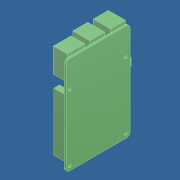
# Autodesk Inventor part: raspberry_pi_4B
Saved by Autodesk Inventor 2022.4 (Build 264492000, 492)
## iProperties
Created: 2023-07-26
Part Number: raspberry_pi_4B
Material: 一般
Document SubType Name: Modeling
Designer: 8326d
Density: 1 g/cm^3
Appearance: 滑らか - 濃い深緑
Author: 8326d
Autodesk Inventor part; units mm, degrees
(part 1 of 2)
ref_plane "YZ Plane" through (0, 0, 0) normal (1, 0, 0) x (0, 1, 0)
ref_plane "XZ Plane" through (0, 0, 0) normal (0, 1, 0) x (-1, 0, 0)
ref_plane "XY Plane" through (0, 0, 0) normal (0, 0, 1) x (1, 0, 0)
sketch "スケッチ1" plane through (0, 0, 0) normal (1, 0, 0) x (0, 1, 0)
  circle A0 centre (61.5, 3.5) radius 3
  circle A1 centre (3.5, 52.5) radius 1.35
  circle A2 centre (3.5, 52.5) radius 3
  circle A3 centre (3.5, 3.5) radius 1.35
  circle A4 centre (3.5, 3.5) radius 3
  circle A5 centre (61.5, 52.5) radius 1.35
  circle A6 centre (61.5, 52.5) radius 3
  circle A7 centre (61.5, 3.5) radius 1.35
  line L0 (3, 0) -> (82, 0)
  arc A8 (82, 0) -> (85, 3) centre (82, 3) ccw
  line L1 (85, 3) -> (85, 53)
  arc A9 (85, 53) -> (82, 56) centre (82, 53) ccw
  line L2 (82, 56) -> (3, 56)
  arc A10 (3, 56) -> (0, 53) centre (3, 53) ccw
  line L3 (0, 53) -> (0, 3)
  arc A11 (0, 3) -> (3, 0) centre (3, 3) ccw
  line L4 (33.225, 5.525) -> (34.375, 5.525)
  line L5 (34.375, 5.525) -> (34.375, 6.675)
  line L6 (34.375, 6.675) -> (33.225, 6.675)
  line L7 (33.225, 6.675) -> (33.225, 5.525)
  arc A12 (33.5, 6.5) -> (33.3, 6.5) centre (33.4, 6.5) ccw
  arc A13 (33.3, 6.5) -> (33.5, 6.5) centre (33.4, 6.5) ccw
  line L8 (6.6, 36.1) -> (17.4, 36.1)
  line L9 (17.4, 36.1) -> (17.4, 49.1)
  line L10 (17.4, 49.1) -> (6.6, 49.1)
  line L11 (6.6, 49.1) -> (6.6, 36.1)
  line L12 (6.8, 36.3) -> (17.2, 36.3)
  line L13 (17.2, 36.3) -> (17.2, 48.9)
  line L14 (17.2, 48.9) -> (6.8, 48.9)
  line L15 (6.8, 48.9) -> (6.8, 36.3)
  line L16 (6.6, 47.9) -> (6.8, 47.9)
  line L17 (6.6, 47.2) -> (6.8, 47.2)
  line L18 (36.4, -0.83) -> (36.4, 6.52)
  line L19 (36.4, 6.52) -> (42.6, 6.52)
  line L20 (42.6, 6.52) -> (42.6, -0.83)
  line L21 (42.6, -0.83) -> (36.4, -0.83)
  line L22 (36.4, -0.83) -> (35.9, -1.33)
  line L23 (35.9, -1.33) -> (35.9, -1.43)
  line L24 (35.9, -1.43) -> (43.1, -1.43)
  line L25 (43.1, -1.43) -> (43.1, -1.33)
  line L26 (43.1, -1.33) -> (42.6, -0.83)
  line L27 (22.9, -0.83) -> (22.9, 6.52)
  line L28 (22.9, 6.52) -> (29.1, 6.52)
  line L29 (29.1, 6.52) -> (29.1, -0.83)
  line L30 (29.1, -0.83) -> (22.9, -0.83)
  line L31 (22.9, -0.83) -> (22.4, -1.33)
  line L32 (22.4, -1.33) -> (22.4, -1.43)
  line L33 (22.4, -1.43) -> (29.6, -1.43)
  line L34 (29.6, -1.43) -> (29.6, -1.33)
  line L35 (29.6, -1.33) -> (29.1, -0.83)
  line L36 (8.95, 48.35) -> (8.15, 48.35)
  line L37 (8.15, 48.35) -> (8.15, 46.75)
  line L38 (8.15, 46.75) -> (8.95, 46.75)
  line L39 (8.95, 46.75) -> (8.95, 48.35)
  line L40 (8.7, 46.85) -> (8.7, 47.15)
  line L41 (8.7, 47.15) -> (8.4, 47.15)
  line L42 (8.4, 47.15) -> (8.4, 46.85)
  line L43 (8.4, 46.85) -> (8.7, 46.85)
  line L44 (68.4, 17.3) -> (68.4, 18.5)
  line L45 (68.4, 18.5) -> (66.4, 18.5)
  line L46 (66.4, 18.5) -> (66.4, 17.3)
  line L47 (66.4, 17.3) -> (68.4, 17.3)
  line L48 (68, 17.3) -> (68, 18.5)
  line L49 (66.8, 17.3) -> (66.8, 18.5)
  line L50 (51.4, 18.6) -> (54.4, 18.6)
  line L51 (54.4, 18.6) -> (54.4, 20.6)
  line L52 (54.4, 20.6) -> (51.4, 20.6)
  line L53 (51.4, 20.6) -> (51.4, 18.6)
  arc A14 (51.8414, 20.3) -> (51.5586, 20.3) centre (51.7, 20.3) ccw
  arc A15 (51.5586, 20.3) -> (51.8414, 20.3) centre (51.7, 20.3) ccw
  line L54 (50.5, 16.9) -> (50.5, 13.9)
  line L55 (50.5, 13.9) -> (52.5, 13.9)
  line L56 (52.5, 13.9) -> (52.5, 16.9)
  line L57 (52.5, 16.9) -> (50.5, 16.9)
  arc A16 (52.3414, 16.6) -> (52.0586, 16.6) centre (52.2, 16.6) ccw
  arc A17 (52.0586, 16.6) -> (52.3414, 16.6) centre (52.2, 16.6) ccw
  line L58 (39.05, 40) -> (39.05, 39.6)
  line L59 (39.05, 39.6) -> (39.45, 40)
  line L60 (39.45, 40) -> (39.05, 40)
  line L61 (39.05, 25) -> (50.55, 25)
  line L62 (50.55, 25) -> (50.55, 40)
  line L63 (50.55, 40) -> (39.05, 40)
  line L64 (39.05, 40) -> (39.05, 25)
  line L65 (68.4, 15.3) -> (68.4, 16.5)
  line L66 (68.4, 16.5) -> (66.4, 16.5)
  line L67 (66.4, 16.5) -> (66.4, 15.3)
  line L68 (66.4, 15.3) -> (68.4, 15.3)
  line L69 (68, 15.3) -> (68, 16.5)
  line L70 (66.8, 15.3) -> (66.8, 16.5)
  line L71 (3.8, 16.3) -> (2.6, 16.3)
  line L72 (2.6, 16.3) -> (2.6, 14.3)
  line L73 (2.6, 14.3) -> (3.8, 14.3)
  line L74 (3.8, 14.3) -> (3.8, 16.3)
  line L75 (3.8, 15.9) -> (2.6, 15.9)
  line L76 (3.8, 14.7) -> (2.6, 14.7)
  line L77 (6.875, -1.25) -> (15.525, -1.25)
  line L78 (15.525, -1.25) -> (15.525, 6.15)
  line L79 (15.525, 6.15) -> (6.875, 6.15)
  line L80 (6.875, 6.15) -> (6.875, -1.25)
  line L81 (12.9, 15.1) -> (12.9, 17.1)
  line L82 (12.9, 17.1) -> (13.9, 18.1)
  line L83 (13.9, 18.1) -> (15.9, 18.1)
  line L84 (15.9, 18.1) -> (16.9, 17.1)
  line L85 (16.9, 17.1) -> (16.9, 15.1)
  line L86 (16.9, 15.1) -> (15.9, 14.1)
  line L87 (15.9, 14.1) -> (13.9, 14.1)
  line L88 (13.9, 14.1) -> (12.9, 15.1)
  line L89 (69.85, 29.75) -> (69.85, 37.05)
  line L90 (69.85, 37.05) -> (65.55, 37.05)
  line L91 (65.55, 37.05) -> (65.55, 29.75)
  line L92 (65.55, 29.75) -> (69.85, 29.75)
  line L93 (68.9, 29.75) -> (68.9, 31.05)
  line L94 (68.9, 31.05) -> (66.5, 31.05)
  line L95 (66.5, 31.05) -> (66.5, 29.75)
  line L96 (68.9, 37.05) -> (68.9, 35.75)
  line L97 (68.9, 35.75) -> (66.5, 35.75)
  line L98 (66.5, 35.75) -> (66.5, 37.05)
  line L99 (65.85, 30.25) -> (66.2, 30.25)
  line L100 (66, 30.05) -> (66, 30.45)
  line L101 (65.85, 30.25) -> (65.8, 30.25)
  line L102 (65.55, 30.75) -> (69.85, 30.75)
  line L103 (69.85, 30.75) -> (69.85, 31.45)
  line L104 (69.85, 31.45) -> (65.55, 31.45)
  line L105 (65.55, 31.45) -> (65.55, 30.75)
  line L106 (88, 37.995) -> (88, 53.505)
  line L107 (88, 53.505) -> (66.65, 53.505)
  line L108 (66.65, 53.505) -> (66.65, 37.995)
  line L109 (66.65, 37.995) -> (88, 37.995)
  line L110 (45.05, 0.3) -> (47.9, 0.3)
  line L111 (47.9, 0.3) -> (47.9, 3.7)
  line L112 (47.9, 3.7) -> (49, 4.8)
  line L113 (49, 4.8) -> (49, 18.2)
  line L114 (49, 18.2) -> (47.85, 19.35)
  line L115 (47.85, 19.35) -> (47.85, 22.7)
  line L116 (47.85, 22.7) -> (45.05, 22.7)
  line L117 (45.05, 22.7) -> (45.05, 0.3)
  line L118 (45.05, 3.5) -> (45.95, 3.5)
  line L119 (45.95, 3.5) -> (45.95, 19.5)
  line L120 (45.95, 19.5) -> (45.05, 19.5)
  line L121 (5.45, 39.2) -> (2.6, 39.2)
  line L122 (2.6, 39.2) -> (2.6, 35.8)
  line L123 (2.6, 35.8) -> (1.5, 34.7)
  line L124 (1.5, 34.7) -> (1.5, 21.3)
  line L125 (1.5, 21.3) -> (2.65, 20.15)
  line L126 (2.65, 20.15) -> (2.65, 16.8)
  line L127 (2.65, 16.8) -> (5.45, 16.8)
  line L128 (5.45, 16.8) -> (5.45, 39.2)
  line L129 (5.45, 36) -> (4.55, 36)
  line L130 (4.55, 36) -> (4.55, 20)
  line L131 (4.55, 20) -> (5.45, 20)
  line L132 (50.5, 0) -> (57.5, 0)
  line L133 (57.5, 0) -> (57.5, 12.5)
  line L134 (57.5, 12.5) -> (50.5, 12.5)
  line L135 (50.5, 12.5) -> (50.5, 0)
  line L136 (51, -2.5) -> (57, -2.5)
  line L137 (57, -2.5) -> (57, 0)
  line L138 (57, 0) -> (51, 0)
  line L139 (51, 0) -> (51, -2.5)
  line L140 (59.9, 18.4) -> (59.9, 16)
  line L141 (59.9, 16) -> (63.1, 16)
  line L142 (63.1, 16) -> (63.1, 18.4)
  line L143 (63.1, 18.4) -> (59.9, 18.4)
  line L144 (59.9, 18.4) -> (59.9, 18.3)
  line L145 (60, 18.3) -> (63, 18.3)
  line L146 (63, 18.3) -> (63, 16.1)
  line L147 (63, 16.1) -> (60, 16.1)
  line L148 (60, 16.1) -> (60, 18.3)
  arc A18 (60.4414, 16.4) -> (60.1586, 16.4) centre (60.3, 16.4) ccw
  arc A19 (60.1586, 16.4) -> (60.4414, 16.4) centre (60.3, 16.4) ccw
  line L149 (2.7, 47.25) -> (2.7, 49.85)
  line L150 (2.7, 49.85) -> (0.1, 49.85)
  line L151 (0.1, 49.85) -> (0.1, 47.25)
  line L152 (0.1, 47.25) -> (2.7, 47.25)
  line L153 (2.7, 48.85) -> (3, 48.85)
  line L154 (3, 48.85) -> (3, 48.25)
  line L155 (3, 48.25) -> (2.7, 48.25)
  arc A20 (2.322, 48.55) -> (0.478, 48.55) centre (1.4, 48.55) ccw
  arc A21 (0.478, 48.55) -> (2.322, 48.55) centre (1.4, 48.55) ccw
  arc A22 (1.6, 48.55) -> (1.2, 48.55) centre (1.4, 48.55) ccw
  arc A23 (1.2, 48.55) -> (1.6, 48.55) centre (1.4, 48.55) ccw
  line L156 (2.3, 47.25) -> (2.3, 47.05)
  line L157 (2.3, 47.05) -> (0.5, 47.05)
  line L158 (0.5, 47.05) -> (0.5, 47.25)
  line L159 (0.5, 49.85) -> (0.5, 50.05)
  line L160 (0.5, 50.05) -> (2.3, 50.05)
  line L161 (2.3, 50.05) -> (2.3, 49.85)
  line L162 (9.05, 43.2) -> (9.05, 42.9)
  line L163 (8.65, 42.9) -> (8.65, 43.2)
  line L164 (8.55, 42.9) -> (9.15, 42.9)
  line L165 (9.15, 42.9) -> (9.15, 43.2)
  line L166 (9.15, 43.2) -> (8.55, 43.2)
  line L167 (8.55, 43.2) -> (8.55, 42.9)
  arc A24 (8.8, 43.05) -> (8.7, 43.05) centre (8.75, 43.05) ccw
  arc A25 (8.7, 43.05) -> (8.8, 43.05) centre (8.75, 43.05) ccw
  line L168 (9.55, 43.8) -> (9.55, 43.5)
  line L169 (9.15, 43.5) -> (9.15, 43.8)
  line L170 (9.05, 43.5) -> (9.65, 43.5)
  line L171 (9.65, 43.5) -> (9.65, 43.8)
  line L172 (9.65, 43.8) -> (9.05, 43.8)
  line L173 (9.05, 43.8) -> (9.05, 43.5)
  arc A26 (9.3, 43.65) -> (9.2, 43.65) centre (9.25, 43.65) ccw
  arc A27 (9.2, 43.65) -> (9.3, 43.65) centre (9.25, 43.65) ccw
  line L174 (8.7, 43.7) -> (8.4, 43.7)
  line L175 (8.4, 44.1) -> (8.7, 44.1)
  line L176 (8.4, 44.2) -> (8.4, 43.6)
  line L177 (8.4, 43.6) -> (8.7, 43.6)
  line L178 (8.7, 43.6) -> (8.7, 44.2)
  line L179 (8.7, 44.2) -> (8.4, 44.2)
  arc A28 (8.6, 44) -> (8.5, 44) centre (8.55, 44) ccw
  arc A29 (8.5, 44) -> (8.6, 44) centre (8.55, 44) ccw
  line L180 (11.95, 44.75) -> (11.65, 44.75)
  line L181 (11.65, 45.15) -> (11.95, 45.15)
  line L182 (11.65, 45.25) -> (11.65, 44.65)
  line L183 (11.65, 44.65) -> (11.95, 44.65)
  line L184 (11.95, 44.65) -> (11.95, 45.25)
  line L185 (11.95, 45.25) -> (11.65, 45.25)
  arc A30 (11.85, 45.05) -> (11.75, 45.05) centre (11.8, 45.05) ccw
  arc A31 (11.75, 45.05) -> (11.85, 45.05) centre (11.8, 45.05) ccw
  line L186 (7.55, 38.35) -> (8.85, 38.35)
  line L187 (8.85, 38.35) -> (8.85, 40.05)
  line L188 (8.85, 40.05) -> (7.55, 40.05)
  line L189 (7.55, 40.05) -> (7.55, 38.35)
  arc A32 (8.05, 39.7) -> (7.65, 39.7) centre (7.85, 39.7) ccw
  arc A33 (7.65, 39.7) -> (8.05, 39.7) centre (7.85, 39.7) ccw
  line L190 (8.15, 46.175) -> (8.275, 46.3)
  line L191 (8.275, 46.3) -> (9.25, 46.3)
  line L192 (9.25, 46.3) -> (9.25, 45.2)
  line L193 (9.25, 45.2) -> (8.15, 45.2)
  line L194 (8.15, 45.2) -> (8.15, 46.175)
  line L195 (88, 2.43) -> (70.3, 2.43)
  line L196 (70.3, 2.43) -> (70.3, 15.57)
  line L197 (70.3, 15.57) -> (88, 15.57)
  line L198 (88, 15.57) -> (88, 1.65)
  line L199 (88, 1.65) -> (87.5, 1.65)
  line L200 (87.5, 1.65) -> (87.5, 2.43)
  line L201 (88, 15.57) -> (88, 16.35)
  line L202 (88, 16.35) -> (87.5, 16.35)
  line L203 (87.5, 16.35) -> (87.5, 15.57)
  line L204 (15.8, 19.5) -> (8.2, 19.5)
  line L205 (8.2, 19.5) -> (8.2, 21.5)
  line L206 (8.2, 21.5) -> (15.8, 21.5)
  line L207 (15.8, 21.5) -> (15.8, 19.5)
  line L208 (62.7, 14.75) -> (62.7, 14.25)
  line L209 (62.7, 14.25) -> (63.7, 14.25)
  line L210 (63.7, 14.25) -> (63.7, 14.75)
  line L211 (63.7, 14.75) -> (62.7, 14.75)
  line L212 (62.95, 14.25) -> (62.95, 14.75)
  line L213 (63.45, 14.25) -> (63.45, 14.75)
  line L214 (38.7, 43.25) -> (38.7, 42.75)
  line L215 (38.7, 42.75) -> (39.7, 42.75)
  line L216 (39.7, 42.75) -> (39.7, 43.25)
  line L217 (39.7, 43.25) -> (38.7, 43.25)
  line L218 (38.95, 42.75) -> (38.95, 43.25)
  line L219 (39.45, 42.75) -> (39.45, 43.25)
  line L220 (52.4, 18.15) -> (52.4, 17.65)
  line L221 (52.4, 17.65) -> (53.4, 17.65)
  line L222 (53.4, 17.65) -> (53.4, 18.15)
  line L223 (53.4, 18.15) -> (52.4, 18.15)
  line L224 (52.65, 17.65) -> (52.65, 18.15)
  line L225 (53.15, 17.65) -> (53.15, 18.15)
  line L226 (56.45, 32.6) -> (56.95, 32.6)
  line L227 (56.95, 32.6) -> (56.95, 33.6)
  line L228 (56.95, 33.6) -> (56.45, 33.6)
  line L229 (56.45, 33.6) -> (56.45, 32.6)
  line L230 (56.95, 32.85) -> (56.45, 32.85)
  line L231 (56.95, 33.35) -> (56.45, 33.35)
  line L232 (10.4, 8.25) -> (10.4, 7.75)
  line L233 (10.4, 7.75) -> (11.4, 7.75)
  line L234 (11.4, 7.75) -> (11.4, 8.25)
  line L235 (11.4, 8.25) -> (10.4, 8.25)
  line L236 (10.65, 7.75) -> (10.65, 8.25)
  line L237 (11.15, 7.75) -> (11.15, 8.25)
  line L238 (8.5, 8.25) -> (8.5, 7.75)
  line L239 (8.5, 7.75) -> (9.5, 7.75)
  line L240 (9.5, 7.75) -> (9.5, 8.25)
  line L241 (9.5, 8.25) -> (8.5, 8.25)
  line L242 (8.75, 7.75) -> (8.75, 8.25)
  line L243 (9.25, 7.75) -> (9.25, 8.25)
  line L244 (67.9, 19.25) -> (67.9, 19.75)
  line L245 (67.9, 19.75) -> (66.9, 19.75)
  line L246 (66.9, 19.75) -> (66.9, 19.25)
  line L247 (66.9, 19.25) -> (67.9, 19.25)
  line L248 (67.65, 19.75) -> (67.65, 19.25)
  line L249 (67.15, 19.75) -> (67.15, 19.25)
  line L250 (66.75, 2.4) -> (67.25, 2.4)
  line L251 (67.25, 2.4) -> (67.25, 3.4)
  line L252 (67.25, 3.4) -> (66.75, 3.4)
  line L253 (66.75, 3.4) -> (66.75, 2.4)
  line L254 (67.25, 2.65) -> (66.75, 2.65)
  line L255 (67.25, 3.15) -> (66.75, 3.15)
  line L256 (69.25, 3.4) -> (68.75, 3.4)
  line L257 (68.75, 3.4) -> (68.75, 2.4)
  line L258 (68.75, 2.4) -> (69.25, 2.4)
  line L259 (69.25, 2.4) -> (69.25, 3.4)
  line L260 (68.75, 3.15) -> (69.25, 3.15)
  line L261 (68.75, 2.65) -> (69.25, 2.65)
  line L262 (67.75, 2.4) -> (68.25, 2.4)
  line L263 (68.25, 2.4) -> (68.25, 3.4)
  line L264 (68.25, 3.4) -> (67.75, 3.4)
  line L265 (67.75, 3.4) -> (67.75, 2.4)
  line L266 (68.25, 2.65) -> (67.75, 2.65)
  line L267 (68.25, 3.15) -> (67.75, 3.15)
  line L268 (57.45, 16.7) -> (56.95, 16.7)
  line L269 (56.95, 16.7) -> (56.95, 15.7)
  line L270 (56.95, 15.7) -> (57.45, 15.7)
  line L271 (57.45, 15.7) -> (57.45, 16.7)
  line L272 (56.95, 16.45) -> (57.45, 16.45)
  line L273 (56.95, 15.95) -> (57.45, 15.95)
  line L274 (57.45, 14.8) -> (56.95, 14.8)
  line L275 (56.95, 14.8) -> (56.95, 13.8)
  line L276 (56.95, 13.8) -> (57.45, 13.8)
  line L277 (57.45, 13.8) -> (57.45, 14.8)
  line L278 (56.95, 14.55) -> (57.45, 14.55)
  line L279 (56.95, 14.05) -> (57.45, 14.05)
  line L280 (62.05, 7.5) -> (62.55, 7.5)
  line L281 (62.55, 7.5) -> (62.55, 8.5)
  line L282 (62.55, 8.5) -> (62.05, 8.5)
  line L283 (62.05, 8.5) -> (62.05, 7.5)
  line L284 (62.55, 7.75) -> (62.05, 7.75)
  line L285 (62.55, 8.25) -> (62.05, 8.25)
  line L286 (54.25, 16.7) -> (53.75, 16.7)
  line L287 (53.75, 16.7) -> (53.75, 15.7)
  line L288 (53.75, 15.7) -> (54.25, 15.7)
  line L289 (54.25, 15.7) -> (54.25, 16.7)
  line L290 (53.75, 16.45) -> (54.25, 16.45)
  line L291 (53.75, 15.95) -> (54.25, 15.95)
  line L292 (54.25, 14.8) -> (53.75, 14.8)
  line L293 (53.75, 14.8) -> (53.75, 13.8)
  line L294 (53.75, 13.8) -> (54.25, 13.8)
  line L295 (54.25, 13.8) -> (54.25, 14.8)
  line L296 (53.75, 14.55) -> (54.25, 14.55)
  line L297 (53.75, 14.05) -> (54.25, 14.05)
  line L298 (62.55, 10.6) -> (62.05, 10.6)
  line L299 (62.05, 10.6) -> (62.05, 9.6)
  line L300 (62.05, 9.6) -> (62.55, 9.6)
  line L301 (62.55, 9.6) -> (62.55, 10.6)
  line L302 (62.05, 10.35) -> (62.55, 10.35)
  line L303 (62.05, 9.85) -> (62.55, 9.85)
  line L304 (69.85, 11) -> (69.35, 11)
  line L305 (69.35, 11) -> (69.35, 10)
  line L306 (69.35, 10) -> (69.85, 10)
  line L307 (69.85, 10) -> (69.85, 11)
  line L308 (69.35, 10.75) -> (69.85, 10.75)
  line L309 (69.35, 10.25) -> (69.85, 10.25)
  line L310 (69.85, 9) -> (69.35, 9)
  line L311 (69.35, 9) -> (69.35, 8)
  line L312 (69.35, 8) -> (69.85, 8)
  line L313 (69.85, 8) -> (69.85, 9)
  line L314 (69.35, 8.75) -> (69.85, 8.75)
  line L315 (69.35, 8.25) -> (69.85, 8.25)
  line L316 (28.75, 23.1) -> (28.25, 23.1)
  line L317 (28.25, 23.1) -> (28.25, 22.1)
  line L318 (28.25, 22.1) -> (28.75, 22.1)
  line L319 (28.75, 22.1) -> (28.75, 23.1)
  line L320 (28.25, 22.85) -> (28.75, 22.85)
  line L321 (28.25, 22.35) -> (28.75, 22.35)
  line L322 (18.2, 48.85) -> (18.2, 48.35)
  line L323 (18.2, 48.35) -> (19.2, 48.35)
  line L324 (19.2, 48.35) -> (19.2, 48.85)
  line L325 (19.2, 48.85) -> (18.2, 48.85)
  line L326 (18.45, 48.35) -> (18.45, 48.85)
  line L327 (18.95, 48.35) -> (18.95, 48.85)
  line L328 (18.2, 47.85) -> (18.2, 47.35)
  line L329 (18.2, 47.35) -> (19.2, 47.35)
  line L330 (19.2, 47.35) -> (19.2, 47.85)
  line L331 (19.2, 47.85) -> (18.2, 47.85)
  line L332 (18.45, 47.35) -> (18.45, 47.85)
  line L333 (18.95, 47.35) -> (18.95, 47.85)
  line L334 (62.5, 35.25) -> (62.5, 34.75)
  line L335 (62.5, 34.75) -> (63.5, 34.75)
  line L336 (63.5, 34.75) -> (63.5, 35.25)
  line L337 (63.5, 35.25) -> (62.5, 35.25)
  line L338 (62.75, 34.75) -> (62.75, 35.25)
  line L339 (63.25, 34.75) -> (63.25, 35.25)
  line L340 (58.9, 31.9) -> (59.4, 31.9)
  line L341 (59.4, 31.9) -> (59.4, 32.9)
  line L342 (59.4, 32.9) -> (58.9, 32.9)
  line L343 (58.9, 32.9) -> (58.9, 31.9)
  line L344 (59.4, 32.15) -> (58.9, 32.15)
  line L345 (59.4, 32.65) -> (58.9, 32.65)
  line L346 (5.6, 12.5) -> (4, 12.5)
  line L347 (4, 12.5) -> (4, 13.3)
  line L348 (4, 13.3) -> (5.6, 13.3)
  line L349 (5.6, 13.3) -> (5.6, 12.5)
  line L350 (5.2, 13.3) -> (5.2, 12.5)
  line L351 (4.3, 13.3) -> (4.3, 12.5)
  line L352 (14.2, 11.9) -> (15.8, 11.9)
  line L353 (15.8, 11.9) -> (15.8, 11.1)
  line L354 (15.8, 11.1) -> (14.2, 11.1)
  line L355 (14.2, 11.1) -> (14.2, 11.9)
  line L356 (14.6, 11.1) -> (14.6, 11.9)
  line L357 (15.5, 11.1) -> (15.5, 11.9)
  line L358 (15.7, 8.5) -> (15.7, 10.1)
  line L359 (15.7, 10.1) -> (16.5, 10.1)
  line L360 (16.5, 10.1) -> (16.5, 8.5)
  line L361 (16.5, 8.5) -> (15.7, 8.5)
  line L362 (16.5, 8.9) -> (15.7, 8.9)
  line L363 (16.5, 9.8) -> (15.7, 9.8)
  line L364 (5.6, 11.1) -> (4, 11.1)
  line L365 (4, 11.1) -> (4, 11.9)
  line L366 (4, 11.9) -> (5.6, 11.9)
  line L367 (5.6, 11.9) -> (5.6, 11.1)
  line L368 (5.2, 11.9) -> (5.2, 11.1)
  line L369 (4.3, 11.9) -> (4.3, 11.1)
  line L370 (14.2, 13.3) -> (15.8, 13.3)
  line L371 (15.8, 13.3) -> (15.8, 12.5)
  line L372 (15.8, 12.5) -> (14.2, 12.5)
  line L373 (14.2, 12.5) -> (14.2, 13.3)
  line L374 (14.6, 12.5) -> (14.6, 13.3)
  line L375 (15.5, 12.5) -> (15.5, 13.3)
  line L376 (7.5, 16.6) -> (9.1, 16.6)
  line L377 (9.1, 16.6) -> (9.1, 15.8)
  line L378 (9.1, 15.8) -> (7.5, 15.8)
  line L379 (7.5, 15.8) -> (7.5, 16.6)
  line L380 (7.9, 15.8) -> (7.9, 16.6)
  line L381 (8.8, 15.8) -> (8.8, 16.6)
  line L382 (61, 33.4) -> (61, 31.8)
  line L383 (61, 31.8) -> (60.2, 31.8)
  line L384 (60.2, 31.8) -> (60.2, 33.4)
  line L385 (60.2, 33.4) -> (61, 33.4)
  line L386 (60.2, 33) -> (61, 33)
  line L387 (60.2, 32.1) -> (61, 32.1)
  line L388 (58.3, 33.4) -> (58.3, 31.8)
  line L389 (58.3, 31.8) -> (57.5, 31.8)
  line L390 (57.5, 31.8) -> (57.5, 33.4)
  line L391 (57.5, 33.4) -> (58.3, 33.4)
  line L392 (57.5, 33) -> (58.3, 33)
  line L393 (57.5, 32.1) -> (58.3, 32.1)
  line L394 (64.7, 8.2) -> (64.7, 9.8)
  line L395 (64.7, 9.8) -> (65.5, 9.8)
  line L396 (65.5, 9.8) -> (65.5, 8.2)
  line L397 (65.5, 8.2) -> (64.7, 8.2)
  line L398 (65.5, 8.6) -> (64.7, 8.6)
  line L399 (65.5, 9.5) -> (64.7, 9.5)
  line L400 (15.05, 41.65) -> (15.05, 41.15)
  line L401 (15.05, 41.15) -> (16.05, 41.15)
  line L402 (16.05, 41.15) -> (16.05, 41.65)
  line L403 (16.05, 41.65) -> (15.05, 41.65)
  line L404 (15.3, 41.15) -> (15.3, 41.65)
  line L405 (15.8, 41.15) -> (15.8, 41.65)
  line L406 (11.85, 38.05) -> (11.35, 38.05)
  line L407 (11.35, 38.05) -> (11.35, 37.05)
  line L408 (11.35, 37.05) -> (11.85, 37.05)
  line L409 (11.85, 37.05) -> (11.85, 38.05)
  line L410 (11.35, 37.8) -> (11.85, 37.8)
  line L411 (11.35, 37.3) -> (11.85, 37.3)
  line L412 (14.4, 38.05) -> (13.9, 38.05)
  line L413 (13.9, 38.05) -> (13.9, 37.05)
  line L414 (13.9, 37.05) -> (14.4, 37.05)
  line L415 (14.4, 37.05) -> (14.4, 38.05)
  line L416 (13.9, 37.8) -> (14.4, 37.8)
  line L417 (13.9, 37.3) -> (14.4, 37.3)
  line L418 (13.55, 38.05) -> (13.05, 38.05)
  line L419 (13.05, 38.05) -> (13.05, 37.05)
  line L420 (13.05, 37.05) -> (13.55, 37.05)
  line L421 (13.55, 37.05) -> (13.55, 38.05)
  line L422 (13.05, 37.8) -> (13.55, 37.8)
  line L423 (13.05, 37.3) -> (13.55, 37.3)
  line L424 (12.7, 38.05) -> (12.2, 38.05)
  line L425 (12.2, 38.05) -> (12.2, 37.05)
  line L426 (12.2, 37.05) -> (12.7, 37.05)
  line L427 (12.7, 37.05) -> (12.7, 38.05)
  line L428 (12.2, 37.8) -> (12.7, 37.8)
  line L429 (12.2, 37.3) -> (12.7, 37.3)
  line L430 (14.8, 37.95) -> (15.3, 37.95)
  line L431 (15.3, 37.95) -> (15.3, 38.95)
  line L432 (15.3, 38.95) -> (14.8, 38.95)
  line L433 (14.8, 38.95) -> (14.8, 37.95)
  line L434 (15.3, 38.2) -> (14.8, 38.2)
  line L435 (15.3, 38.7) -> (14.8, 38.7)
  line L436 (10.05, 44.4) -> (10.05, 44.9)
  line L437 (10.05, 44.9) -> (9.05, 44.9)
  line L438 (9.05, 44.9) -> (9.05, 44.4)
  line L439 (9.05, 44.4) -> (10.05, 44.4)
  line L440 (9.8, 44.9) -> (9.8, 44.4)
  line L441 (9.3, 44.9) -> (9.3, 44.4)
  line L442 (12.55, 8.4) -> (12.05, 8.4)
  line L443 (12.05, 8.4) -> (12.05, 7.4)
  line L444 (12.05, 7.4) -> (12.55, 7.4)
  line L445 (12.55, 7.4) -> (12.55, 8.4)
  line L446 (12.05, 8.15) -> (12.55, 8.15)
  line L447 (12.05, 7.65) -> (12.55, 7.65)
  line L448 (11.2, 44.75) -> (10.9, 44.75)
  line L449 (10.9, 45.15) -> (11.2, 45.15)
  line L450 (10.9, 45.25) -> (10.9, 44.65)
  line L451 (10.9, 44.65) -> (11.2, 44.65)
  line L452 (11.2, 44.65) -> (11.2, 45.25)
  line L453 (11.2, 45.25) -> (10.9, 45.25)
  line L454 (10.75, 48.05) -> (10.75, 48.35)
  line L455 (11.15, 48.35) -> (11.15, 48.05)
  line L456 (11.25, 48.35) -> (10.65, 48.35)
  line L457 (10.65, 48.35) -> (10.65, 48.05)
  line L458 (10.65, 48.05) -> (11.25, 48.05)
  line L459 (11.25, 48.05) -> (11.25, 48.35)
  line L460 (3.15, 42.4) -> (2.85, 42.4)
  line L461 (2.85, 42.8) -> (3.15, 42.8)
  line L462 (2.85, 42.9) -> (2.85, 42.3)
  line L463 (2.85, 42.3) -> (3.15, 42.3)
  line L464 (3.15, 42.3) -> (3.15, 42.9)
  line L465 (3.15, 42.9) -> (2.85, 42.9)
  line L466 (3.15, 41.1) -> (2.85, 41.1)
  line L467 (2.85, 41.5) -> (3.15, 41.5)
  line L468 (2.85, 41.6) -> (2.85, 41)
  line L469 (2.85, 41) -> (3.15, 41)
  line L470 (3.15, 41) -> (3.15, 41.6)
  line L471 (3.15, 41.6) -> (2.85, 41.6)
  line L472 (0.8, 42.4) -> (0.5, 42.4)
  line L473 (0.5, 42.8) -> (0.8, 42.8)
  line L474 (0.5, 42.9) -> (0.5, 42.3)
  line L475 (0.5, 42.3) -> (0.8, 42.3)
  line L476 (0.8, 42.3) -> (0.8, 42.9)
  line L477 (0.8, 42.9) -> (0.5, 42.9)
  line L478 (0.8, 41.1) -> (0.5, 41.1)
  line L479 (0.5, 41.5) -> (0.8, 41.5)
  line L480 (0.5, 41.6) -> (0.5, 41)
  line L481 (0.5, 41) -> (0.8, 41)
  line L482 (0.8, 41) -> (0.8, 41.6)
  line L483 (0.8, 41.6) -> (0.5, 41.6)
  line L484 (5.2475, 47.8146) -> (5.0354, 47.6025)
  line L485 (4.7525, 47.8854) -> (4.9646, 48.0975)
  line L486 (4.6818, 47.9561) -> (5.1061, 47.5318)
  line L487 (5.1061, 47.5318) -> (5.3182, 47.7439)
  line L488 (5.3182, 47.7439) -> (4.8939, 48.1682)
  line L489 (4.8939, 48.1682) -> (4.6818, 47.9561)
  line L490 (10.55, 46) -> (10.25, 46)
  line L491 (10.25, 46.4) -> (10.55, 46.4)
  line L492 (10.25, 46.5) -> (10.25, 45.9)
  line L493 (10.25, 45.9) -> (10.55, 45.9)
  line L494 (10.55, 45.9) -> (10.55, 46.5)
  line L495 (10.55, 46.5) -> (10.25, 46.5)
  line L496 (9.6, 46.65) -> (9.9, 46.65)
  line L497 (9.9, 46.25) -> (9.6, 46.25)
  line L498 (9.9, 46.15) -> (9.9, 46.75)
  line L499 (9.9, 46.75) -> (9.6, 46.75)
  line L500 (9.6, 46.75) -> (9.6, 46.15)
  line L501 (9.6, 46.15) -> (9.9, 46.15)
  line L502 (10.2, 45.45) -> (10.2, 45.15)
  line L503 (9.8, 45.15) -> (9.8, 45.45)
  line L504 (9.7, 45.15) -> (10.3, 45.15)
  line L505 (10.3, 45.15) -> (10.3, 45.45)
  line L506 (10.3, 45.45) -> (9.7, 45.45)
  line L507 (9.7, 45.45) -> (9.7, 45.15)
  line L508 (10.1, 47.65) -> (10.4, 47.65)
  line L509 (10.4, 47.25) -> (10.1, 47.25)
  line L510 (10.4, 47.15) -> (10.4, 47.75)
  line L511 (10.4, 47.75) -> (10.1, 47.75)
  line L512 (10.1, 47.75) -> (10.1, 47.15)
  line L513 (10.1, 47.15) -> (10.4, 47.15)
  line L514 (11.85, 47.5) -> (12.15, 47.5)
  line L515 (12.15, 47.1) -> (11.85, 47.1)
  line L516 (12.15, 47) -> (12.15, 47.6)
  line L517 (12.15, 47.6) -> (11.85, 47.6)
  line L518 (11.85, 47.6) -> (11.85, 47)
  line L519 (11.85, 47) -> (12.15, 47)
  line L520 (12.45, 46.4) -> (12.45, 46.1)
  line L521 (12.05, 46.1) -> (12.05, 46.4)
  line L522 (11.95, 46.1) -> (12.55, 46.1)
  line L523 (12.55, 46.1) -> (12.55, 46.4)
  line L524 (12.55, 46.4) -> (11.95, 46.4)
  line L525 (11.95, 46.4) -> (11.95, 46.1)
  line L526 (10.8025, 47.1854) -> (11.0146, 47.3975)
  line L527 (11.2975, 47.1146) -> (11.0854, 46.9025)
  line L528 (11.3682, 47.0439) -> (10.9439, 47.4682)
  line L529 (10.9439, 47.4682) -> (10.7318, 47.2561)
  line L530 (10.7318, 47.2561) -> (11.1561, 46.8318)
  line L531 (11.1561, 46.8318) -> (11.3682, 47.0439)
  line L532 (7.6, 45.4) -> (7.3, 45.4)
  line L533 (7.3, 45.8) -> (7.6, 45.8)
  line L534 (7.3, 45.9) -> (7.3, 45.3)
  line L535 (7.3, 45.3) -> (7.6, 45.3)
  line L536 (7.6, 45.3) -> (7.6, 45.9)
  line L537 (7.6, 45.9) -> (7.3, 45.9)
  line L538 (7.6, 42.85) -> (7.3, 42.85)
  line L539 (7.3, 43.25) -> (7.6, 43.25)
  line L540 (7.3, 43.35) -> (7.3, 42.75)
  line L541 (7.3, 42.75) -> (7.6, 42.75)
  line L542 (7.6, 42.75) -> (7.6, 43.35)
  line L543 (7.6, 43.35) -> (7.3, 43.35)
  line L544 (7.8, 44.65) -> (8.1, 44.65)
  line L545 (8.1, 44.25) -> (7.8, 44.25)
  line L546 (8.1, 44.15) -> (8.1, 44.75)
  line L547 (8.1, 44.75) -> (7.8, 44.75)
  line L548 (7.8, 44.75) -> (7.8, 44.15)
  line L549 (7.8, 44.15) -> (8.1, 44.15)
  line L550 (62.9626, 39.0303) -> (64.7303, 37.2626)
  line L551 (64.7303, 37.2626) -> (65.4374, 37.9697)
  line L552 (65.4374, 37.9697) -> (63.6697, 39.7374)
  line L553 (63.6697, 39.7374) -> (62.9626, 39.0303)
  arc A34 (63.3161, 39.0303) -> (63.1747, 39.0304) centre (63.2454, 39.0303) ccw
  arc A35 (63.1747, 39.0304) -> (63.3161, 39.0303) centre (63.2454, 39.0303) ccw
  line L554 (62.9626, 42.3303) -> (64.7303, 40.5626)
  line L555 (64.7303, 40.5626) -> (65.4374, 41.2697)
  line L556 (65.4374, 41.2697) -> (63.6697, 43.0374)
  line L557 (63.6697, 43.0374) -> (62.9626, 42.3303)
  arc A36 (63.3161, 42.3303) -> (63.1747, 42.3304) centre (63.2454, 42.3303) ccw
  arc A37 (63.1747, 42.3304) -> (63.3161, 42.3303) centre (63.2454, 42.3303) ccw
  line L558 (30.05, 21.95) -> (30.05, 21.35)
  line L559 (30.05, 21.35) -> (30.35, 21.35)
  line L560 (30.35, 21.35) -> (30.35, 21.95)
  line L561 (30.35, 21.95) -> (30.05, 21.95)
  line L562 (30.05, 21.85) -> (30.35, 21.85)
  line L563 (30.35, 21.45) -> (30.05, 21.45)
  line L564 (36.2939, 43.0818) -> (36.7182, 43.5061)
  line L565 (36.7182, 43.5061) -> (36.5061, 43.7182)
  line L566 (36.5061, 43.7182) -> (36.0818, 43.2939)
  line L567 (36.0818, 43.2939) -> (36.2939, 43.0818)
  line L568 (36.3646, 43.1525) -> (36.1525, 43.3646)
  line L569 (36.4354, 43.6475) -> (36.6475, 43.4354)
  line L570 (62.5, 35.85) -> (63.1, 35.85)
  line L571 (63.1, 35.85) -> (63.1, 36.15)
  line L572 (63.1, 36.15) -> (62.5, 36.15)
  line L573 (62.5, 36.15) -> (62.5, 35.85)
  line L574 (62.6, 35.85) -> (62.6, 36.15)
  line L575 (63, 36.15) -> (63, 35.85)
  line L576 (65.1, 19.35) -> (65.7, 19.35)
  line L577 (65.7, 19.35) -> (65.7, 19.65)
  line L578 (65.7, 19.65) -> (65.1, 19.65)
  line L579 (65.1, 19.65) -> (65.1, 19.35)
  line L580 (65.2, 19.35) -> (65.2, 19.65)
  line L581 (65.6, 19.65) -> (65.6, 19.35)
  line L582 (1.85, 17.4) -> (1.85, 18)
  line L583 (1.85, 18) -> (1.55, 18)
  line L584 (1.55, 18) -> (1.55, 17.4)
  line L585 (1.55, 17.4) -> (1.85, 17.4)
  line L586 (1.85, 17.5) -> (1.55, 17.5)
  line L587 (1.55, 17.9) -> (1.85, 17.9)
  line L588 (38.55, 41.8) -> (39.15, 41.8)
  line L589 (39.15, 41.8) -> (39.15, 42.1)
  line L590 (39.15, 42.1) -> (38.55, 42.1)
  line L591 (38.55, 42.1) -> (38.55, 41.8)
  line L592 (38.65, 41.8) -> (38.65, 42.1)
  line L593 (39.05, 42.1) -> (39.05, 41.8)
  line L594 (22.2, 41) -> (21.6, 41)
  line L595 (21.6, 41) -> (21.6, 40.7)
  line L596 (21.6, 40.7) -> (22.2, 40.7)
  line L597 (22.2, 40.7) -> (22.2, 41)
  line L598 (22.1, 41) -> (22.1, 40.7)
  line L599 (21.7, 40.7) -> (21.7, 41)
  line L600 (22.2, 41.65) -> (21.6, 41.65)
  line L601 (21.6, 41.65) -> (21.6, 41.35)
  line L602 (21.6, 41.35) -> (22.2, 41.35)
  line L603 (22.2, 41.35) -> (22.2, 41.65)
  line L604 (22.1, 41.65) -> (22.1, 41.35)
  line L605 (21.7, 41.35) -> (21.7, 41.65)
  line L606 (44.3, 40.85) -> (43.7, 40.85)
  line L607 (43.7, 40.85) -> (43.7, 40.55)
  line L608 (43.7, 40.55) -> (44.3, 40.55)
  line L609 (44.3, 40.55) -> (44.3, 40.85)
  line L610 (44.2, 40.85) -> (44.2, 40.55)
  line L611 (43.8, 40.55) -> (43.8, 40.85)
  line L612 (45.3, 40.55) -> (45.9, 40.55)
  line L613 (45.9, 40.55) -> (45.9, 40.85)
  line L614 (45.9, 40.85) -> (45.3, 40.85)
  line L615 (45.3, 40.85) -> (45.3, 40.55)
  line L616 (45.4, 40.55) -> (45.4, 40.85)
  line L617 (45.8, 40.85) -> (45.8, 40.55)
  line L618 (55.45, 14.3) -> (55.45, 13.7)
  line L619 (55.45, 13.7) -> (55.75, 13.7)
  line L620 (55.75, 13.7) -> (55.75, 14.3)
  line L621 (55.75, 14.3) -> (55.45, 14.3)
  line L622 (55.45, 14.2) -> (55.75, 14.2)
  line L623 (55.75, 13.8) -> (55.45, 13.8)
  line L624 (33.5, 3.15) -> (32.9, 3.15)
  line L625 (32.9, 3.15) -> (32.9, 2.85)
  line L626 (32.9, 2.85) -> (33.5, 2.85)
  line L627 (33.5, 2.85) -> (33.5, 3.15)
  line L628 (33.4, 3.15) -> (33.4, 2.85)
  line L629 (33, 2.85) -> (33, 3.15)
  line L630 (32.6, 7.7) -> (32, 7.7)
  line L631 (32, 7.7) -> (32, 7.4)
  line L632 (32, 7.4) -> (32.6, 7.4)
  line L633 (32.6, 7.4) -> (32.6, 7.7)
  line L634 (32.5, 7.7) -> (32.5, 7.4)
  line L635 (32.1, 7.4) -> (32.1, 7.7)
  line L636 (65.35, 6.5) -> (65.35, 5.9)
  line L637 (65.35, 5.9) -> (65.65, 5.9)
  line L638 (65.65, 5.9) -> (65.65, 6.5)
  line L639 (65.65, 6.5) -> (65.35, 6.5)
  line L640 (65.35, 6.4) -> (65.65, 6.4)
  line L641 (65.65, 6) -> (65.35, 6)
  line L642 (56.15, 14.3) -> (56.15, 13.7)
  line L643 (56.15, 13.7) -> (56.45, 13.7)
  line L644 (56.45, 13.7) -> (56.45, 14.3)
  line L645 (56.45, 14.3) -> (56.15, 14.3)
  line L646 (56.15, 14.2) -> (56.45, 14.2)
  line L647 (56.45, 13.8) -> (56.15, 13.8)
  line L648 (54.75, 14.3) -> (54.75, 13.7)
  line L649 (54.75, 13.7) -> (55.05, 13.7)
  line L650 (55.05, 13.7) -> (55.05, 14.3)
  line L651 (55.05, 14.3) -> (54.75, 14.3)
  line L652 (54.75, 14.2) -> (55.05, 14.2)
  line L653 (55.05, 13.8) -> (54.75, 13.8)
  line L654 (26.2182, 47.0939) -> (25.7939, 47.5182)
  line L655 (25.7939, 47.5182) -> (25.5818, 47.3061)
  line L656 (25.5818, 47.3061) -> (26.0061, 46.8818)
  line L657 (26.0061, 46.8818) -> (26.2182, 47.0939)
  line L658 (26.1475, 47.1646) -> (25.9354, 46.9525)
  line L659 (25.6525, 47.2354) -> (25.8646, 47.4475)
  line L660 (7.55, 8.4) -> (7.55, 7.8)
  line L661 (7.55, 7.8) -> (7.85, 7.8)
  line L662 (7.85, 7.8) -> (7.85, 8.4)
  line L663 (7.85, 8.4) -> (7.55, 8.4)
  line L664 (7.55, 8.3) -> (7.85, 8.3)
  line L665 (7.85, 7.9) -> (7.55, 7.9)
  line L666 (59.35, 16.9) -> (59.35, 17.5)
  line L667 (59.35, 17.5) -> (59.05, 17.5)
  line L668 (59.05, 17.5) -> (59.05, 16.9)
  line L669 (59.05, 16.9) -> (59.35, 16.9)
  line L670 (59.35, 17) -> (59.05, 17)
  line L671 (59.05, 17.4) -> (59.35, 17.4)
  line L672 (63.65, 17.5) -> (63.65, 16.9)
  line L673 (63.65, 16.9) -> (63.95, 16.9)
  line L674 (63.95, 16.9) -> (63.95, 17.5)
  line L675 (63.95, 17.5) -> (63.65, 17.5)
  line L676 (63.65, 17.4) -> (63.95, 17.4)
  line L677 (63.95, 17) -> (63.65, 17)
  line L678 (7.55, 42.25) -> (7.55, 41.65)
  line L679 (7.55, 41.65) -> (7.85, 41.65)
  line L680 (7.85, 41.65) -> (7.85, 42.25)
  line L681 (7.85, 42.25) -> (7.55, 42.25)
  line L682 (7.55, 42.15) -> (7.85, 42.15)
  line L683 (7.85, 41.75) -> (7.55, 41.75)
  line L684 (15.8, 42.05) -> (16.4, 42.05)
  line L685 (16.4, 42.05) -> (16.4, 42.35)
  line L686 (16.4, 42.35) -> (15.8, 42.35)
  line L687 (15.8, 42.35) -> (15.8, 42.05)
  line L688 (15.9, 42.05) -> (15.9, 42.35)
  line L689 (16.3, 42.35) -> (16.3, 42.05)
  line L690 (9.85, 38.4) -> (9.85, 37.8)
  line L691 (9.85, 37.8) -> (10.15, 37.8)
  line L692 (10.15, 37.8) -> (10.15, 38.4)
  line L693 (10.15, 38.4) -> (9.85, 38.4)
  line L694 (9.85, 38.3) -> (10.15, 38.3)
  line L695 (10.15, 37.9) -> (9.85, 37.9)
  line L696 (14.8, 43.1) -> (15.4, 43.1)
  line L697 (15.4, 43.1) -> (15.4, 43.4)
  line L698 (15.4, 43.4) -> (14.8, 43.4)
  line L699 (14.8, 43.4) -> (14.8, 43.1)
  line L700 (14.9, 43.1) -> (14.9, 43.4)
  line L701 (15.3, 43.4) -> (15.3, 43.1)
  line L702 (13.75, 44.8) -> (13.75, 45.4)
  line L703 (13.75, 45.4) -> (13.45, 45.4)
  line L704 (13.45, 45.4) -> (13.45, 44.8)
  line L705 (13.45, 44.8) -> (13.75, 44.8)
  line L706 (13.75, 44.9) -> (13.45, 44.9)
  line L707 (13.45, 45.3) -> (13.75, 45.3)
  line L708 (13.15, 44.8) -> (13.15, 45.4)
  line L709 (13.15, 45.4) -> (12.85, 45.4)
  line L710 (12.85, 45.4) -> (12.85, 44.8)
  line L711 (12.85, 44.8) -> (13.15, 44.8)
  line L712 (13.15, 44.9) -> (12.85, 44.9)
  line L713 (12.85, 45.3) -> (13.15, 45.3)
  line L714 (53.4, 25.35) -> (54, 25.35)
  line L715 (54, 25.35) -> (54, 25.65)
  line L716 (54, 25.65) -> (53.4, 25.65)
  line L717 (53.4, 25.65) -> (53.4, 25.35)
  line L718 (53.5, 25.35) -> (53.5, 25.65)
  line L719 (53.9, 25.65) -> (53.9, 25.35)
  line L720 (53.4, 25.95) -> (54, 25.95)
  line L721 (54, 25.95) -> (54, 26.25)
  line L722 (54, 26.25) -> (53.4, 26.25)
  line L723 (53.4, 26.25) -> (53.4, 25.95)
  line L724 (53.5, 25.95) -> (53.5, 26.25)
  line L725 (53.9, 26.25) -> (53.9, 25.95)
  line L726 (53.4, 22.95) -> (54, 22.95)
  line L727 (54, 22.95) -> (54, 23.25)
  line L728 (54, 23.25) -> (53.4, 23.25)
  line L729 (53.4, 23.25) -> (53.4, 22.95)
  line L730 (53.5, 22.95) -> (53.5, 23.25)
  line L731 (53.9, 23.25) -> (53.9, 22.95)
  line L732 (53.4, 23.55) -> (54, 23.55)
  line L733 (54, 23.55) -> (54, 23.85)
  line L734 (54, 23.85) -> (53.4, 23.85)
  line L735 (53.4, 23.85) -> (53.4, 23.55)
  line L736 (53.5, 23.55) -> (53.5, 23.85)
  line L737 (53.9, 23.85) -> (53.9, 23.55)
  line L738 (65.7, 25.05) -> (65.1, 25.05)
  line L739 (65.1, 25.05) -> (65.1, 24.75)
  line L740 (65.1, 24.75) -> (65.7, 24.75)
  line L741 (65.7, 24.75) -> (65.7, 25.05)
  line L742 (65.6, 25.05) -> (65.6, 24.75)
  line L743 (65.2, 24.75) -> (65.2, 25.05)
  line L744 (65.7, 24.4) -> (65.1, 24.4)
  line L745 (65.1, 24.4) -> (65.1, 24.1)
  line L746 (65.1, 24.1) -> (65.7, 24.1)
  line L747 (65.7, 24.1) -> (65.7, 24.4)
  line L748 (65.6, 24.4) -> (65.6, 24.1)
  line L749 (65.2, 24.1) -> (65.2, 24.4)
  line L750 (65.7, 21.45) -> (65.1, 21.45)
  line L751 (65.1, 21.45) -> (65.1, 21.15)
  line L752 (65.1, 21.15) -> (65.7, 21.15)
  line L753 (65.7, 21.15) -> (65.7, 21.45)
  line L754 (65.6, 21.45) -> (65.6, 21.15)
  line L755 (65.2, 21.15) -> (65.2, 21.45)
  line L756 (65.7, 20.8) -> (65.1, 20.8)
  line L757 (65.1, 20.8) -> (65.1, 20.5)
  line L758 (65.1, 20.5) -> (65.7, 20.5)
  line L759 (65.7, 20.5) -> (65.7, 20.8)
  line L760 (65.6, 20.8) -> (65.6, 20.5)
  line L761 (65.2, 20.5) -> (65.2, 20.8)
  line L762 (9.3, 41.85) -> (8.7, 41.85)
  line L763 (8.7, 41.85) -> (8.7, 41.55)
  line L764 (8.7, 41.55) -> (9.3, 41.55)
  line L765 (9.3, 41.55) -> (9.3, 41.85)
  line L766 (9.2, 41.85) -> (9.2, 41.55)
  line L767 (8.8, 41.55) -> (8.8, 41.85)
  line L768 (12.55, 44.8) -> (12.55, 45.4)
  line L769 (12.55, 45.4) -> (12.25, 45.4)
  line L770 (12.25, 45.4) -> (12.25, 44.8)
  line L771 (12.25, 44.8) -> (12.55, 44.8)
  line L772 (12.55, 44.9) -> (12.25, 44.9)
  line L773 (12.25, 45.3) -> (12.55, 45.3)
  line L774 (8.5, 38) -> (7.9, 38)
  line L775 (7.9, 38) -> (7.9, 37.7)
  line L776 (7.9, 37.7) -> (8.5, 37.7)
  line L777 (8.5, 37.7) -> (8.5, 38)
  line L778 (8.4, 38) -> (8.4, 37.7)
  line L779 (8, 37.7) -> (8, 38)
  line L780 (8.2, 40.7) -> (7.6, 40.7)
  line L781 (7.6, 40.7) -> (7.6, 40.4)
  line L782 (7.6, 40.4) -> (8.2, 40.4)
  line L783 (8.2, 40.4) -> (8.2, 40.7)
  line L784 (8.1, 40.7) -> (8.1, 40.4)
  line L785 (7.7, 40.4) -> (7.7, 40.7)
  line L786 (15.15, 40.1) -> (15.75, 40.1)
  line L787 (15.75, 40.1) -> (15.75, 40.4)
  line L788 (15.75, 40.4) -> (15.15, 40.4)
  line L789 (15.15, 40.4) -> (15.15, 40.1)
  line L790 (15.25, 40.1) -> (15.25, 40.4)
  line L791 (15.65, 40.4) -> (15.65, 40.1)
  line L792 (9.65, 42.5) -> (9.05, 42.5)
  line L793 (9.05, 42.5) -> (9.05, 42.2)
  line L794 (9.05, 42.2) -> (9.65, 42.2)
  line L795 (9.65, 42.2) -> (9.65, 42.5)
  line L796 (9.55, 42.5) -> (9.55, 42.2)
  line L797 (9.15, 42.2) -> (9.15, 42.5)
  line L798 (53.4, 24.15) -> (54, 24.15)
  line L799 (54, 24.15) -> (54, 24.45)
  line L800 (54, 24.45) -> (53.4, 24.45)
  line L801 (53.4, 24.45) -> (53.4, 24.15)
  line L802 (53.5, 24.15) -> (53.5, 24.45)
  line L803 (53.9, 24.45) -> (53.9, 24.15)
  line L804 (53.4, 24.75) -> (54, 24.75)
  line L805 (54, 24.75) -> (54, 25.05)
  line L806 (54, 25.05) -> (53.4, 25.05)
  line L807 (53.4, 25.05) -> (53.4, 24.75)
  line L808 (53.5, 24.75) -> (53.5, 25.05)
  line L809 (53.9, 25.05) -> (53.9, 24.75)
  line L810 (16.55, 38.9) -> (16.55, 37.3)
  line L811 (16.55, 37.3) -> (15.75, 37.3)
  line L812 (15.75, 37.3) -> (15.75, 38.9)
  line L813 (15.75, 38.9) -> (16.55, 38.9)
  line L814 (15.75, 38.5) -> (16.55, 38.5)
  line L815 (15.75, 37.6) -> (16.55, 37.6)
  line L816 (64, 12.4) -> (64, 11.6)
  line L817 (64, 11.6) -> (62.4, 11.6)
  line L818 (62.4, 11.6) -> (62.4, 12.4)
  line L819 (62.4, 12.4) -> (64, 12.4)
  line L820 (64.1, 12.5) -> (64.1, 11.5)
  line L821 (64.1, 11.5) -> (62.3, 11.5)
  line L822 (62.3, 11.5) -> (62.3, 12.5)
  line L823 (62.3, 12.5) -> (64.1, 12.5)
  line L824 (63.8, 12.5) -> (63.8, 12.9)
  line L825 (63.8, 12.9) -> (63.6, 12.9)
  line L826 (63.6, 12.9) -> (63.6, 12.5)
  line L827 (63.6, 12.5) -> (62.8, 12.5)
  line L828 (62.8, 12.5) -> (62.8, 12.9)
  line L829 (62.8, 12.9) -> (62.6, 12.9)
  line L830 (62.6, 12.9) -> (62.6, 12.5)
  line L831 (63.3, 11.5) -> (63.3, 11.1)
  line L832 (63.3, 11.1) -> (63.1, 11.1)
  line L833 (63.1, 11.1) -> (63.1, 11.5)
  line L834 (0.75, 10.7) -> (0.75, 12.3)
  line L835 (0.75, 12.3) -> (1.45, 12.3)
  line L836 (1.45, 12.3) -> (1.45, 10.7)
  line L837 (1.45, 10.7) -> (0.75, 10.7)
  line L838 (1.1, 11.3) -> (1.4, 11.6)
  line L839 (1.4, 11.6) -> (0.8, 11.6)
  line L840 (0.8, 11.6) -> (1.1, 11.3)
  line L841 (1.1, 11.3) -> (1.1, 11)
  line L842 (0.8, 11.3) -> (1.4, 11.3)
  line L843 (1.1, 11.6) -> (1.1, 12)
  line L844 (1.45, 10.9) -> (0.75, 10.9)
  line L845 (1.45, 12.1) -> (0.75, 12.1)
  line L846 (0.75, 12.15) -> (0.45, 12.15)
  line L847 (0.45, 12.15) -> (0.35, 12.05)
  line L848 (0.35, 12.05) -> (0.35, 10.95)
  line L849 (88, 33.57) -> (88, 20.43)
  line L850 (0.45, 10.85) -> (0.75, 10.85)
  line L851 (0.75, 7.1) -> (0.75, 8.7)
  line L852 (0.75, 8.7) -> (1.45, 8.7)
  line L853 (1.45, 8.7) -> (1.45, 7.1)
  line L854 (1.45, 7.1) -> (0.75, 7.1)
  line L855 (1.1, 7.7) -> (1.4, 8)
  line L856 (1.4, 8) -> (0.8, 8)
  line L857 (0.8, 8) -> (1.1, 7.7)
  line L858 (1.1, 7.7) -> (1.1, 7.4)
  line L859 (0.8, 7.7) -> (1.4, 7.7)
  line L860 (1.1, 8) -> (1.1, 8.4)
  line L861 (1.45, 7.3) -> (0.75, 7.3)
  line L862 (1.45, 8.5) -> (0.75, 8.5)
  line L863 (0.75, 8.55) -> (0.45, 8.55)
  line L864 (0.45, 8.55) -> (0.35, 8.45)
  line L865 (0.35, 8.45) -> (0.35, 7.35)
  line L866 (0.35, 7.35) -> (0.45, 7.25)
  line L867 (0.45, 7.25) -> (0.75, 7.25)
  line L868 (6.7, 17.1) -> (9.5, 17.1)
  line L869 (9.5, 17.1) -> (9.5, 19.1)
  line L870 (9.5, 19.1) -> (6.7, 19.1)
  line L871 (6.7, 19.1) -> (6.7, 17.1)
  line L872 (6.2, 17.5) -> (7.15, 17.5)
  line L873 (7.15, 17.5) -> (7.15, 18.7)
  line L874 (7.15, 18.7) -> (6.2, 18.7)
  line L875 (6.2, 18.7) -> (6.2, 17.5)
  line L876 (10, 17.5) -> (9.05, 17.5)
  line L877 (9.05, 17.5) -> (9.05, 18.7)
  line L878 (9.05, 18.7) -> (10, 18.7)
  line L879 (10, 18.7) -> (10, 17.5)
  line L880 (7.3, 19.1) -> (7.3, 17.1)
  line L881 (7.3, 17.1) -> (7.5, 17.1)
  line L882 (7.5, 17.1) -> (7.5, 19.1)
  line L883 (7.5, 19.1) -> (7.3, 19.1)
  line L884 (21.8, 10.7) -> (21.8, 6.3)
  line L885 (21.8, 6.3) -> (18.2, 6.3)
  line L886 (18.2, 6.3) -> (18.2, 10.7)
  line L887 (18.2, 10.7) -> (21.8, 10.7)
  line L888 (20.9, 10.7) -> (20.9, 11)
  line L889 (20.9, 11) -> (19.1, 11)
  line L890 (19.1, 11) -> (19.1, 10.7)
  line L891 (20.9, 6.3) -> (20.9, 6)
  line L892 (20.9, 6) -> (19.1, 6)
  line L893 (19.1, 6) -> (19.1, 6.3)
  line L894 (21.8, 10.1) -> (18.2, 10.1)
  line L895 (18.2, 10.1) -> (18.2, 9.8)
  line L896 (18.2, 9.8) -> (21.8, 9.8)
  line L897 (21.8, 9.8) -> (21.8, 10.1)
  line L898 (32.4, 1.5) -> (32.4, 4.5)
  line L899 (32.4, 4.5) -> (30.8, 4.5)
  line L900 (30.8, 4.5) -> (30.8, 1.5)
  line L901 (30.8, 1.5) -> (32.4, 1.5)
  line L902 (32.3, 1.6) -> (32.3, 4.4)
  line L903 (32.3, 4.4) -> (30.9, 4.4)
  line L904 (30.9, 4.4) -> (30.9, 1.6)
  line L905 (30.9, 1.6) -> (32.3, 1.6)
  line L906 (32.4, 1.8) -> (33, 1.8)
  line L907 (33, 1.8) -> (33, 2.3)
  line L908 (33, 2.3) -> (32.4, 2.3)
  line L909 (32.4, 3.7) -> (33, 3.7)
  line L910 (33, 3.7) -> (33, 4.2)
  line L911 (33, 4.2) -> (32.4, 4.2)
  line L912 (30.8, 2.75) -> (30.2, 2.75)
  line L913 (30.2, 2.75) -> (30.2, 3.25)
  line L914 (30.2, 3.25) -> (30.8, 3.25)
  line L915 (60.5, 11.5) -> (60.5, 14.5)
  line L916 (60.5, 14.5) -> (58.9, 14.5)
  line L917 (58.9, 14.5) -> (58.9, 11.5)
  line L918 (58.9, 11.5) -> (60.5, 11.5)
  line L919 (60.4, 11.6) -> (60.4, 14.4)
  line L920 (60.4, 14.4) -> (59, 14.4)
  line L921 (59, 14.4) -> (59, 11.6)
  line L922 (59, 11.6) -> (60.4, 11.6)
  line L923 (60.5, 11.8) -> (61.1, 11.8)
  line L924 (61.1, 11.8) -> (61.1, 12.3)
  line L925 (61.1, 12.3) -> (60.5, 12.3)
  line L926 (60.5, 13.7) -> (61.1, 13.7)
  line L927 (61.1, 13.7) -> (61.1, 14.2)
  line L928 (61.1, 14.2) -> (60.5, 14.2)
  line L929 (58.9, 12.75) -> (58.3, 12.75)
  line L930 (58.3, 12.75) -> (58.3, 13.25)
  line L931 (58.3, 13.25) -> (58.9, 13.25)
  line L932 (67.2, 7.15) -> (67.2, 4.25)
  line L933 (67.2, 4.25) -> (68.8, 4.25)
  line L934 (68.8, 4.25) -> (68.8, 7.15)
  line L935 (68.8, 7.15) -> (67.2, 7.15)
  line L936 (67.3, 7.05) -> (67.3, 4.35)
  line L937 (67.3, 4.35) -> (68.7, 4.35)
  line L938 (68.7, 4.35) -> (68.7, 7.05)
  line L939 (68.7, 7.05) -> (67.3, 7.05)
  line L940 (67.2, 6.85) -> (66.6, 6.85)
  line L941 (66.6, 6.85) -> (66.6, 6.45)
  line L942 (66.6, 6.45) -> (67.2, 6.45)
  line L943 (67.2, 5.9) -> (66.6, 5.9)
  line L944 (66.6, 5.9) -> (66.6, 5.5)
  line L945 (66.6, 5.5) -> (67.2, 5.5)
  line L946 (67.2, 4.95) -> (66.6, 4.95)
  line L947 (66.6, 4.95) -> (66.6, 4.55)
  line L948 (66.6, 4.55) -> (67.2, 4.55)
  line L949 (68.8, 6.85) -> (69.4, 6.85)
  line L950 (69.4, 6.85) -> (69.4, 6.45)
  line L951 (69.4, 6.45) -> (68.8, 6.45)
  line L952 (68.8, 4.95) -> (69.4, 4.95)
  line L953 (69.4, 4.95) -> (69.4, 4.55)
  line L954 (69.4, 4.55) -> (68.8, 4.55)
  line L955 (68.8, 5.9) -> (69.4, 5.9)
  line L956 (69.4, 5.9) -> (69.4, 5.5)
  line L957 (69.4, 5.5) -> (68.8, 5.5)
  arc A38 (67.7414, 6.7) -> (67.4586, 6.7) centre (67.6, 6.7) ccw
  arc A39 (67.4586, 6.7) -> (67.7414, 6.7) centre (67.6, 6.7) ccw
  line L958 (56.6, 16.9) -> (54.6, 16.9)
  line L959 (54.6, 16.9) -> (54.6, 15.7)
  line L960 (54.6, 15.7) -> (56.6, 15.7)
  line L961 (56.6, 15.7) -> (56.6, 16.9)
  line L962 (56.5, 16.8) -> (54.7, 16.8)
  line L963 (54.7, 16.8) -> (54.7, 15.8)
  line L964 (54.7, 15.8) -> (56.5, 15.8)
  line L965 (56.5, 15.8) -> (56.5, 16.8)
  line L966 (56.375, 16.9) -> (56.375, 17.375)
  line L967 (56.375, 17.375) -> (56.125, 17.375)
  line L968 (56.125, 17.375) -> (56.125, 16.9)
  line L969 (55.725, 16.9) -> (55.725, 17.375)
  line L970 (55.725, 17.375) -> (55.475, 17.375)
  line L971 (55.475, 17.375) -> (55.475, 16.9)
  line L972 (55.075, 16.9) -> (55.075, 17.375)
  line L973 (55.075, 17.375) -> (54.825, 17.375)
  line L974 (54.825, 17.375) -> (54.825, 16.9)
  line L975 (56.125, 15.225) -> (56.125, 15.7)
  line L976 (56.375, 15.7) -> (56.375, 15.225)
  line L977 (56.375, 15.225) -> (56.125, 15.225)
  line L978 (55.725, 15.7) -> (55.725, 15.225)
  line L979 (55.725, 15.225) -> (55.475, 15.225)
  line L980 (55.075, 15.7) -> (55.075, 15.225)
  line L981 (55.075, 15.225) -> (54.825, 15.225)
  line L982 (54.825, 15.225) -> (54.825, 15.7)
  line L983 (55.475, 15.225) -> (55.475, 15.7)
  line L984 (14.435, 44.135) -> (9.965, 44.135)
  line L985 (9.965, 44.135) -> (9.965, 38.865)
  line L986 (9.965, 38.865) -> (14.3004, 38.865)
  line L987 (14.3004, 38.865) -> (14.435, 38.9996)
  line L988 (14.435, 38.9996) -> (14.435, 44.135)
  line L989 (63.5, 28) -> (55.5, 28)
  line L990 (55.5, 28) -> (55.5, 20)
  line L991 (55.5, 20) -> (63.5, 20)
  line L992 (63.5, 20) -> (63.5, 28)
  arc A40 (63.141, 27.5) -> (62.859, 27.5) centre (63, 27.5) ccw
  arc A41 (62.859, 27.5) -> (63.141, 27.5) centre (63, 27.5) ccw
  line L993 (0.35, 10.95) -> (0.45, 10.85)
  line L994 (55.5, 41) -> (61.5, 41)
  line L995 (61.5, 41) -> (61.5, 35)
  line L996 (61.5, 35) -> (55.5, 35)
  arc A42 (56.6414, 35.5) -> (56.3586, 35.5) centre (56.5, 35.5) ccw
  arc A43 (56.3586, 35.5) -> (56.6414, 35.5) centre (56.5, 35.5) ccw
  line L997 (12.2, 18.1) -> (11, 18.1)
  line L998 (11, 18.1) -> (11, 16.1)
  line L999 (11, 16.1) -> (12.2, 16.1)
  line L1000 (12.2, 16.1) -> (12.2, 18.1)
  line L1001 (12.2, 17.7) -> (11, 17.7)
  line L1002 (12.2, 16.5) -> (11, 16.5)
  line L1003 (52.3, 31.4) -> (51.1, 31.4)
  line L1004 (51.1, 31.4) -> (51.1, 29.4)
  line L1005 (51.1, 29.4) -> (52.3, 29.4)
  line L1006 (52.3, 29.4) -> (52.3, 31.4)
  line L1007 (52.3, 31) -> (51.1, 31)
  line L1008 (52.3, 29.8) -> (51.1, 29.8)
  line L1009 (47.5, 41.8) -> (47.5, 40.6)
  line L1010 (47.5, 40.6) -> (49.5, 40.6)
  line L1011 (49.5, 40.6) -> (49.5, 41.8)
  line L1012 (49.5, 41.8) -> (47.5, 41.8)
  line L1013 (47.9, 41.8) -> (47.9, 40.6)
  line L1014 (49.1, 41.8) -> (49.1, 40.6)
  line L1015 (68.8, 14.3) -> (67.6, 14.3)
  line L1016 (67.6, 14.3) -> (67.6, 12.3)
  line L1017 (67.6, 12.3) -> (68.8, 12.3)
  line L1018 (68.8, 12.3) -> (68.8, 14.3)
  line L1019 (68.8, 13.9) -> (67.6, 13.9)
  line L1020 (68.8, 12.7) -> (67.6, 12.7)
  line L1021 (60.7, 9.5) -> (60.7, 10.7)
  line L1022 (60.7, 10.7) -> (58.7, 10.7)
  line L1023 (58.7, 10.7) -> (58.7, 9.5)
  line L1024 (58.7, 9.5) -> (60.7, 9.5)
  line L1025 (60.3, 9.5) -> (60.3, 10.7)
  line L1026 (59.1, 9.5) -> (59.1, 10.7)
  line L1027 (60.7, 7.4) -> (60.7, 8.6)
  line L1028 (60.7, 8.6) -> (58.7, 8.6)
  line L1029 (58.7, 8.6) -> (58.7, 7.4)
  line L1030 (58.7, 7.4) -> (60.7, 7.4)
  line L1031 (60.3, 7.4) -> (60.3, 8.6)
  line L1032 (59.1, 7.4) -> (59.1, 8.6)
  line L1033 (63.2001, 33.85) -> (61.9999, 33.85)
  line L1034 (61.9999, 33.85) -> (61.9999, 31.85)
  line L1035 (61.9999, 31.85) -> (63.2001, 31.85)
  line L1036 (63.2001, 31.85) -> (63.2001, 33.85)
  line L1037 (63.2, 33.45) -> (62, 33.45)
  line L1038 (63.2, 32.25) -> (62, 32.25)
  line L1039 (18.8, 16.9) -> (17.6, 16.9)
  line L1040 (17.6, 16.9) -> (17.6, 14.9)
  line L1041 (17.6, 14.9) -> (18.8, 14.9)
  line L1042 (18.8, 14.9) -> (18.8, 16.9)
  line L1043 (18.8, 16.5) -> (17.6, 16.5)
  line L1044 (18.8, 15.3) -> (17.6, 15.3)
  line L1045 (20.7, 16.9) -> (19.5, 16.9)
  line L1046 (19.5, 16.9) -> (19.5, 14.9)
  line L1047 (19.5, 14.9) -> (20.7, 14.9)
  line L1048 (20.7, 14.9) -> (20.7, 16.9)
  line L1049 (20.7, 16.5) -> (19.5, 16.5)
  line L1050 (20.7, 15.3) -> (19.5, 15.3)
  line L1051 (2.6, 8.15) -> (3.8, 8.15)
  line L1052 (3.8, 8.15) -> (3.8, 10.15)
  line L1053 (3.8, 10.15) -> (2.6, 10.15)
  line L1054 (2.6, 10.15) -> (2.6, 8.15)
  line L1055 (2.6, 8.55) -> (3.8, 8.55)
  line L1056 (2.6, 9.75) -> (3.8, 9.75)
  line L1057 (66.9, 12.05) -> (66.9, 14.55)
  line L1058 (66.9, 14.55) -> (64.9, 14.55)
  line L1059 (64.9, 14.55) -> (64.9, 12.05)
  line L1060 (64.9, 12.05) -> (66.9, 12.05)
  line L1061 (64.9, 12.75) -> (66.9, 12.75)
  line L1062 (64.9, 13.85) -> (66.9, 13.85)
  line L1063 (4.5, 10.45) -> (4.5, 7.95)
  line L1064 (4.5, 7.95) -> (6.5, 7.95)
  line L1065 (6.5, 7.95) -> (6.5, 10.45)
  line L1066 (6.5, 10.45) -> (4.5, 10.45)
  line L1067 (6.5, 9.75) -> (4.5, 9.75)
  line L1068 (6.5, 8.65) -> (4.5, 8.65)
  line L1069 (13.1, 10.45) -> (13.1, 7.95)
  line L1070 (13.1, 7.95) -> (15.1, 7.95)
  line L1071 (15.1, 7.95) -> (15.1, 10.45)
  line L1072 (15.1, 10.45) -> (13.1, 10.45)
  line L1073 (15.1, 9.75) -> (13.1, 9.75)
  line L1074 (15.1, 8.65) -> (13.1, 8.65)
  line L1075 (6.5, 14.05) -> (6.5, 16.55)
  line L1076 (6.5, 16.55) -> (4.5, 16.55)
  line L1077 (4.5, 16.55) -> (4.5, 14.05)
  line L1078 (4.5, 14.05) -> (6.5, 14.05)
  line L1079 (4.5, 14.75) -> (6.5, 14.75)
  line L1080 (4.5, 15.85) -> (6.5, 15.85)
  line L1081 (68.95, 10.3) -> (66.05, 10.3)
  line L1082 (66.05, 10.3) -> (66.05, 8.7)
  line L1083 (66.05, 8.7) -> (68.95, 8.7)
  line L1084 (68.95, 8.7) -> (68.95, 10.3)
  line L1085 (68.85, 10.2) -> (66.15, 10.2)
  line L1086 (66.15, 10.2) -> (66.15, 8.8)
  line L1087 (66.15, 8.8) -> (68.85, 8.8)
  line L1088 (68.85, 8.8) -> (68.85, 10.2)
  line L1089 (68.65, 10.3) -> (68.65, 10.9)
  line L1090 (68.65, 10.9) -> (68.25, 10.9)
  line L1091 (68.25, 10.9) -> (68.25, 10.3)
  line L1092 (67.7, 10.3) -> (67.7, 10.9)
  line L1093 (67.7, 10.9) -> (67.3, 10.9)
  line L1094 (67.3, 10.9) -> (67.3, 10.3)
  line L1095 (66.75, 10.3) -> (66.75, 10.9)
  line L1096 (66.75, 10.9) -> (66.35, 10.9)
  line L1097 (66.35, 10.9) -> (66.35, 10.3)
  line L1098 (68.65, 8.7) -> (68.65, 8.1)
  line L1099 (68.65, 8.1) -> (68.25, 8.1)
  line L1100 (68.25, 8.1) -> (68.25, 8.7)
  line L1101 (66.75, 8.7) -> (66.75, 8.1)
  line L1102 (66.75, 8.1) -> (66.35, 8.1)
  line L1103 (66.35, 8.1) -> (66.35, 8.7)
  line L1104 (7.4, 9.7) -> (7.4, 14.7)
  line L1105 (7.4, 14.7) -> (12.4, 14.7)
  line L1106 (12.4, 14.7) -> (12.4, 9.7)
  line L1107 (12.4, 9.7) -> (7.4, 9.7)
  arc A44 (7.85, 10.05) -> (7.65, 10.05) centre (7.75, 10.05) ccw
  arc A45 (7.65, 10.05) -> (7.85, 10.05) centre (7.75, 10.05) ccw
  line L1108 (36.75, 25) -> (36.75, 40)
  line L1109 (36.75, 40) -> (21.75, 40)
  line L1110 (21.75, 40) -> (21.75, 25.506)
  line L1111 (21.75, 25.506) -> (22.256, 25)
  line L1112 (22.256, 25) -> (36.75, 25)
  line L1113 (59, 43.86) -> (64, 43.86)
  line L1114 (64, 43.86) -> (64, 48.86)
  line L1115 (64, 48.86) -> (59, 48.86)
  line L1116 (59, 48.86) -> (59, 43.86)